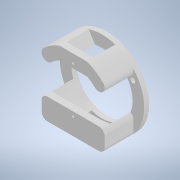
# Autodesk Inventor part: Soporte_Servo
Saved by Autodesk Inventor 2020.1 (Build 241239000, 239)
## iProperties
Created: 2019-12-05
Part Number: Soporte_Servo
Material: Generic
Document SubType Name: Modeling
Designer: Daniel
Density: 1 g/cm^3
Appearance: Default
Author: Daniel
Autodesk Inventor part; units mm, degrees
ref_plane "YZ Plane" through (0, 0, 0) normal (1, 0, 0) x (0, 1, 0)
ref_plane "XZ Plane" through (0, 0, 0) normal (0, 1, 0) x (-1, 0, 0)
sketch "Sketch1" plane through (0, 0, 0) normal (0, 0, 1) x (1, 0, 0)
  circle A0 centre (-21.5, 0) radius 1.25 projected
  circle A1 centre (21.5, 0) radius 1.25 projected
  circle A2 centre (0, 21.5) radius 1.25 projected
  circle A3 centre (0, -21.5) radius 1.25 projected
  circle A4 centre (0, 0) radius 25.5 projected
  circle A5 centre (0, 0) radius 17.5 projected
  circle A6 centre (0, 0) radius 18.5
  circle A7 centre (0, -21.5) radius 1.45
  circle A8 centre (18.6195, 10.75) radius 1.45
  circle A9 centre (-18.6195, 10.75) radius 1.45
  dimension "d0" = 1
  dimension "d28" = 0.2
  dimension "d31" = 360
  constraints: 4 centre point, 2 coincident, 7 other
  measures "d0" radial gap between concentric circles of A5 A6
  measures "d28" radial gap between concentric circles of A7 A3
extrude "Extrusion1" add sketch "Sketch1" along normal blind 3 contours A0 | A1 | A2 | A4
sketch "Sketch2" plane through (0, 0, 3) normal (0, 0, 1) x (1, 0, 0)
  circle A0 centre (0, 21.5) radius 1.45 construction
  line L0 (0, 0) -> (15.5563, 15.5563) construction
  line L1 (0, 0) -> (38.5383, 0) construction
  circle A1 centre (0, 0) radius 25.5 projected
  line L2 (-25.5, 0) -> (-18.5, 0) construction
  circle A2 centre (0, 0) radius 18.5 projected
  circle A3 centre (0, 0) radius 22 construction
  circle A4 centre (15.5563, 15.5563) radius 3.5
  circle A5 centre (-15.5563, 15.5563) radius 3.5
  circle A6 centre (-15.5563, -15.5563) radius 3.5
  circle A7 centre (15.5563, -15.5563) radius 3.5
  dimension "d9" = 44
  dimension "d8" = 45
  dimension "d12" = 360
  constraints: 6 end point, 4 centre point, 3 coincident, 2 horizontal, 2 horizontal alignment, 14 other
  measures "d8" angle of L1 L0
extrude "Extrusion2" add sketch "Sketch2" along normal blind 17.45 contours A4 | A7 | A5 | A6
sketch "Sketch3" plane through (15.5563, 15.5563, 20.45) normal (0, 0, 1) x (1, 0, 0)
  line L0 (-10.3063, -21.6563) -> (-20.8063, -21.6563) projected
  line L1 (-20.8063, 0.8437) -> (-10.3063, 0.8437) projected
  arc A0 (-28.6378, -2.4749) -> (-33.5876, 2.4749) centre (-31.1127, 0) ccw projected
  line L2 (-27.7159, 0.8437) -> (-3.3968, 0.8437)
  line L3 (3.5, -21.6563) -> (-34.6127, -21.6563)
  line L4 (3.5, -21.6563) -> (3.5, -31.1127)
  line L5 (0, -34.6127) -> (-31.1127, -34.6127)
  line L6 (-34.6127, -31.1127) -> (-34.6127, -21.6563)
  circle A1 centre (0, -31.1127) radius 3.5 projected
  circle A2 centre (-31.1127, -31.1127) radius 3.5 projected
  circle A3 centre (0, -31.1127) radius 3.5 projected
  circle A4 centre (-31.1127, -31.1127) radius 3.5 projected
  line L7 (3.5, 0) -> (3.5, 8.6437)
  line L8 (3.5, 8.6437) -> (-34.6127, 8.6437)
  line L9 (-34.6127, 8.6437) -> (-34.6127, 0)
  circle A5 centre (-31.1127, 0) radius 3.5 projected
  circle A6 centre (0, 0) radius 3.5 projected
  line L10 (-20.8063, 5.6437) -> (-16.1063, 5.6437) projected
  point P0 (-15.5563, -15.5563)
  point P1 (0, -34.6127)
  point P2 (-10.3063, 0.8437)
  dimension "d16" = 3
  constraints: 16 end point, 8 point on circle, 5 tangent, 4 perpendicular, 2 collinear, 2 horizontal, 2 vertical
  measures "d16" distance between parallel lines of L8 L10
extrude "Extrusion3" add sketch "Sketch3" against normal blind 4
fillet "Fillet1" radius 3.5 4 edges at (19.0563, 24.2, 18.45) (19.0563, -6.1, 18.45) (-19.0563, -6.1, 18.45) (-19.0563, 24.2, 18.45)
sketch "Sketch4" plane through (15.5563, 15.5563, 16.45) normal (0, 0, -1) x (-1, 0, 0)
  circle A0 centre (15.5563, 3.4937) radius 2.4 projected
  circle A1 centre (15.5563, -24.3063) radius 2.4 projected
  point P0 (15.5563, -15.5563)
  constraints: 2 coincident
hole "Hole1" at (0, -8.75, 16.45) at (0, 19.05, 16.45) direction (0, 0, 1) diameter 1.2 depth 10 tip angle 118
sketch "Sketch5" plane through (0, 0, 3) normal (0, 0, 1) x (1, 0, 0)
  arc A0 (18.0312, 18.0312) -> (13.0815, 13.0815) centre (15.5563, 15.5563) ccw projected
  arc A1 (18.0312, 18.0312) -> (-18.0312, 18.0312) centre (0, 0) ccw projected
  arc A2 (-13.0815, 13.0815) -> (-18.0312, 18.0312) centre (-15.5563, 15.5563) ccw projected
  arc A3 (13.0815, 13.0815) -> (-13.0815, 13.0815) centre (0, 0) ccw projected
  circle A4 centre (0, 19.05) radius 0.6 projected
  arc A5 (-15.5563, 24.2) -> (-19.0563, 20.7) centre (-15.5563, 20.7) ccw projected
  line L0 (-19.0563, 20.7) -> (-19.0563, 15.5563) projected
  arc A6 (-19.0563, 15.5563) -> (-12.1595, 16.4) centre (-15.5563, 15.5563) ccw projected
  line L1 (-12.1595, 16.4) -> (12.1595, 16.4) projected
  arc A7 (12.1595, 16.4) -> (19.0563, 15.5563) centre (15.5563, 15.5563) ccw projected
  line L2 (19.0563, 15.5563) -> (19.0563, 20.7) projected
  arc A8 (19.0563, 20.7) -> (15.5563, 24.2) centre (15.5563, 20.7) ccw projected
  line L3 (15.5563, 24.2) -> (-15.5563, 24.2) projected
  arc A9 (18.0312, 18.0312) -> (-18.0312, 18.0312) centre (0, 0) ccw projected
  line L4 (8.038, 24.2) -> (4.1382, 18.0312)
  arc A10 (13.0815, 13.0815) -> (-13.0815, 13.0815) centre (0, 0) ccw projected
  line L5 (-8.038, 24.2) -> (-4.1382, 18.0312)
  point P0 (8.038, 24.2)
  point P1 (-8.038, 24.2)
  point P2 (-0.2363, 18.4985)
  point P3 (0.2363, 18.4985)
  point P4 (-12.1595, 16.4)
  point P5 (-8.561, 16.4)
  point P6 (8.038, 24.2)
  constraints: 4 end point, 4 point on circle, 2 point on line
extrude "Extrusion4" add sketch "Sketch5" along normal up to surface (17.45 mm away) contours A0 L1 A3 L4 A1 | A0 A3 L1 | L5 A3 L1 A2 A1 | A3 A2 L1
sketch "Sketch6" plane through (15.5563, 15.5563, 16.45) normal (0, 0, -1) x (-1, 0, 0)
  arc A0 (7.5183, 8.6437) -> (-2.4749, 2.4749) centre (15.5563, -15.5563) ccw projected
  line L0 (7.5183, 8.6437) -> (0, 8.6437) projected
  arc A1 (0, 8.6437) -> (-3.5, 5.1437) centre (0, 5.1437) ccw projected
  line L1 (-3.5, 5.1437) -> (-3.5, 0) projected
  arc A2 (-2.4749, 2.4749) -> (-3.5, 0) centre (0, 0) ccw projected
  arc A3 (33.5876, 2.4749) -> (23.5944, 8.6437) centre (15.5563, -15.5563) ccw projected
  arc A4 (34.6127, 0) -> (33.5876, 2.4749) centre (31.1127, 0) ccw projected
  line L2 (34.6127, 0) -> (34.6127, 5.1437) projected
  arc A5 (34.6127, 5.1437) -> (31.1127, 8.6437) centre (31.1127, 5.1437) ccw projected
  line L3 (31.1127, 8.6437) -> (23.5944, 8.6437) projected
extrude "Extrusion5" cut sketch "Sketch6" against normal blind 10
sketch "Sketch7" plane through (0, 0, 3) normal (0, 0, 1) x (1, 0, 0)
  circle A0 centre (0, -21.5) radius 1.45 projected
  arc A1 (13.0815, -13.0815) -> (18.0312, -18.0312) centre (15.5563, -15.5563) ccw projected
  arc A2 (-13.0815, -13.0815) -> (13.0815, -13.0815) centre (0, 0) ccw projected
  arc A3 (-18.0312, -18.0312) -> (-13.0815, -13.0815) centre (-15.5563, -15.5563) ccw projected
  arc A4 (-18.0312, -18.0312) -> (18.0312, -18.0312) centre (0, 0) ccw projected
  arc A5 (18.0312, -18.0312) -> (13.0815, -13.0815) centre (15.5563, -15.5563) ccw projected
  arc A6 (18.0312, -18.0312) -> (18.0312, 18.0312) centre (0, 0) ccw projected
  arc A7 (13.0815, 13.0815) -> (18.0312, 18.0312) centre (15.5563, 15.5563) ccw projected
  arc A8 (13.0815, -13.0815) -> (13.0815, 13.0815) centre (0, 0) ccw projected
  circle A9 centre (18.6195, 10.75) radius 1.45 projected
  arc A10 (-13.0815, -13.0815) -> (-18.0312, -18.0312) centre (-15.5563, -15.5563) ccw projected
  arc A11 (-13.0815, 13.0815) -> (-13.0815, -13.0815) centre (0, 0) ccw projected
  arc A12 (-18.0312, 18.0312) -> (-13.0815, 13.0815) centre (-15.5563, 15.5563) ccw projected
  arc A13 (-18.0312, 18.0312) -> (-18.0312, -18.0312) centre (0, 0) ccw projected
  circle A14 centre (-18.6195, 10.75) radius 1.45 projected
  circle A15 centre (0, -8.75) radius 0.6 projected
  arc A16 (-15.5563, -6.1) -> (-19.0563, -9.6) centre (-15.5563, -9.6) ccw projected
  line L0 (-19.0563, -9.6) -> (-19.0563, -15.5563) projected
  arc A17 (-19.0563, -15.5563) -> (-15.5563, -19.0563) centre (-15.5563, -15.5563) ccw projected
  line L1 (-15.5563, -19.0563) -> (15.5563, -19.0563) projected
  arc A18 (15.5563, -19.0563) -> (19.0563, -15.5563) centre (15.5563, -15.5563) ccw projected
  line L2 (19.0563, -15.5563) -> (19.0563, -9.6) projected
  arc A19 (19.0563, -9.6) -> (15.5563, -6.1) centre (15.5563, -9.6) ccw projected
  line L3 (15.5563, -6.1) -> (-15.5563, -6.1) projected
  arc A20 (-13.0815, -13.0815) -> (13.0815, -13.0815) centre (0, 0) ccw projected
  line L4 (-6.3274, -17.3843) -> (-8.7215, -23.9622)
  arc A21 (-18.0312, -18.0312) -> (18.0312, -18.0312) centre (0, 0) ccw projected
  line L5 (6.3274, -17.3843) -> (8.7215, -23.9622)
  line L6 (0, -21.5) -> (0, -25.5) construction
  point P0 (6.9359, -19.0563)
  point P1 (15.5563, -19.0563)
  point P2 (17.2966, -6.5633)
  point P3 (-6.9359, -19.0563)
  point P4 (-13.0815, -13.0815)
  point P5 (-13.0815, -13.0815)
  point P6 (-13.0815, -13.0815)
  point P7 (-13.0815, -13.0815)
  point P8 (-17.2966, -6.5633)
  dimension "d37" = 40
  dimension "d38" = 20
  constraints: 6 end point, 5 point on circle, 2 line through centre
  measures "d37" angle of L4 L5
  measures "d38" angle of L6 L5
extrude "Extrusion6" add sketch "Sketch7" along normal up to surface (17.45 mm away) contours A1 L1 L5 A2 | A8 A19 L2 A5 | L4 L1 A3 A2 | A10 L0 A16 A11
ref_plane "Work Plane1" through (15.5563, -19.0563, 3) normal (-0.7465912, -0.665283, 0) x (0, 0, 1)
sketch "Sketch8" plane through (15.5563, -19.0563, 3) normal (-0.7465912, -0.665283, 0) x (0, 0, 1)
  line L0 (13.45, 6.1073) -> (13.45, 17.354) projected
  line L1 (13.45, 17.354) -> (17.45, 17.354) projected
  line L2 (17.45, 17.354) -> (17.45, 0) projected
  line L3 (17.45, 0) -> (0, 0) projected
  line L4 (0, 0) -> (0, -0.9011) projected
  line L5 (0, -0.9011) -> (-3, -0.9011) projected
  line L6 (-3, -0.9011) -> (-3, 6.1073) projected
  line L7 (-3, 6.1073) -> (13.45, 6.1073) projected
  line L8 (17.45, 50.0545) -> (17.45, 43.0461) projected
  line L9 (17.45, 43.0461) -> (0, 43.0461) projected
  line L10 (0, 43.0461) -> (-3, 43.0461) projected
  line L11 (-3, 43.0461) -> (-3, 50.0545) projected
  line L12 (-3, 50.0545) -> (17.45, 50.0545) projected
  line L13 (13.45, 14.5573) -> (5, 6.1073)
  point P0 (-3, 24.5767)
  dimension "d41" = 8
  dimension "d49" = 45
  constraints: 2 end point, 2 point on line
  measures "d41" distance of L13.end L6.end
  measures "d49" angle of L7 L13
extrude "Extrusion7" add sketch "Sketch8" along normal blind 1 and the other way blind 2 contours L7 L13 L0
mirror "Mirror1" about plane through (0, 0, 0) normal (1, 0, 0) of "Extrusion7"
body "Solid1"
